# Autodesk Inventor part: JUMPER-PAD-3-NC_BY_PASTE
Saved by Autodesk Inventor 2016 SP1 (Build 200210100, 210)
## iProperties
Created: 2015-11-19
Part Number: JUMPER-PAD-3-NC_BY_PASTE
Material: Generic
Document SubType Name: Modeling
Designer: PhillipD
Density: 1 g/cm^3
Appearance: PAD-JUMPER-3-NC_BY_PASTE_YES_SILK_FULL_BOX, JUMPER-PAD-3-NC_BY_PASTE
Author: PhillipD
Autodesk Inventor part; units mm, degrees
ref_plane "YZ Plane" through (0, 0, 0) normal (1, 0, 0) x (0, 1, 0)
ref_plane "XZ Plane" through (0, 0, 0) normal (0, 1, 0) x (-1, 0, 0)
ref_plane "XY Plane" through (0, 0, 0) normal (0, 0, 1) x (1, 0, 0)
sketch3d "PAD-JUMPER-3-NC_BY_PASTE_YES_SILK_FULL_BOX, JUMPER-PAD-3-NC_"
  constraints: 8 end point
sketch "PAD-JUMPER-3-NC_BY_PASTE_YES_SILK_FULL_BOX, JUMPER-PAD-3-NC_BY_PASTE_52" plane through (0, 0, 0) normal (0, 0, 1) x (1, 0, 0)
  line L0 (-1.524, 1.016) -> (1.524, 1.016)
  line L1 (1.524, 1.016) -> (1.524, -1.0922)
  line L2 (1.524, -1.0922) -> (-1.524, -1.0922)
  line L3 (-1.524, -1.0922) -> (-1.524, 1.016)
extrude "Extrusion1" add sketch "PAD-JUMPER-3-NC_BY_PASTE_YES_SILK_FULL_BOX, JUMPER-PAD-3-NC_BY_PASTE_52" along normal blind 1
body "Solid1"
